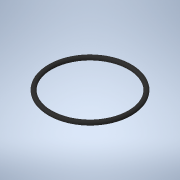
# Autodesk Inventor part: pneu_com_piso
Saved by Autodesk Inventor 2021 (Build 250183000, 183)
## iProperties
Created: 2020-05-19
Part Number: pneu_com_piso
Material: Genérico
Document SubType Name: Modeling
Designer: Mathe
Density: 1.05269 g/cm^3
Appearance: Rubber - Black
Mass: 2.1 g
Surface Area: 22.7988 cm^2
Volume: 1.99489 cm^3
Author: Mathe
Autodesk Inventor part; units mm, degrees
ref_plane "XZ Plane" through (0, 0, 0) normal (0, 1, 0) x (-1, 0, 0)
ref_plane "XY Plane" through (0, 0, 0) normal (0, 0, 1) x (1, 0, 0)
sketch "Esboço1" plane through (0, 0, 0) normal (0, 0, 1) x (1, 0, 0)
  line L0 (0, 0) -> (33, 0)
  circle A0 centre (33, 0) radius 1.75
  line L1 (0, 0) -> (0, 10)
  dimension "d0" = 33
  dimension "d1" = 3.5
  dimension "d2" = 10
  constraints: 4 end point, 1 centre point, 1 coincident, 1 horizontal
  measures "d0" distance of L0.start L0.end
  measures "d1" diameter of A0
  measures "d2" distance of L0.start L1.end
revolve "Revolução1" add sketch "Esboço1" angle 360 about axis through (0, 0, 0) along (0, 1, 0)
ref_plane "Plano de trabalho2" through (34.75, 0, 0) normal (1, 0, 0) x (0, 1, 0)
mirror "Mirror1" about plane through (0, 0, 0) normal (1, 0, 0)
ref_plane "Work Plane3" through (-34.75, 0, 0) normal (1, 0, 0) x (0, 1, 0)
